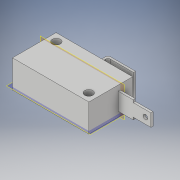
# Autodesk Inventor part: game-switch
Saved by Autodesk Inventor 2017 (Build 210142000, 142)
## iProperties
Created: 2017-02-21
Part Number: game-switch
Material: Generic
Document SubType Name: Modeling
Designer: John
Density: 1 g/cm^3
Appearance: Default
Author: John
Autodesk Inventor part; units mm, degrees
ref_plane "YZ Plane" through (0, 0, 0) normal (1, 0, 0) x (0, 1, 0)
ref_plane "XZ Plane" through (0, 0, 0) normal (0, 1, 0) x (-1, 0, 0)
sketch "Sketch1" plane through (0, 0, 0) normal (0, 1, 0) x (-1, 0, 0)
  line L0 (0, 0) -> (-28, 0)
  line L1 (-28, 0) -> (-28, 16)
  line L2 (-28, 16) -> (0, 16)
  line L3 (0, 16) -> (0, 0)
  circle A0 centre (-25.1, 13.15) radius 1.5
  circle A1 centre (-2.9, 2.85) radius 1.5
  line L4 (-28, 8) -> (0, 8) construction
  line L5 (-14, 0) -> (-14, 16) construction
  line L6 (-25.1, 13.15) -> (-28, 13.15) construction
  line L7 (-25.1, 13.15) -> (-25.1, 16) construction
  line L8 (-2.9, 2.85) -> (-2.9, 0) construction
  line L9 (-2.9, 2.85) -> (0, 2.85) construction
  dimension "d0" = 28
  dimension "d1" = 16
  dimension "d2" = 3
  dimension "d3" = 3
  dimension "d4" = 22.2
  dimension "d5" = 10.3
  constraints: 20 end point, 5 perpendicular, 4 midpoint, 4 parallel, 4 point on line, 2 centre point, 1 horizontal
  measures "d0" distance of L1.end L2.end
  measures "d1" distance of L0.end L1.end
  measures "d2" diameter of A0
  measures "d3" diameter of A1
  measures "d4" horizontal distance of L6.start L8.start
  measures "d5" vertical distance of L8.start L6.start
extrude "Extrusion1" add sketch "Sketch1" along normal blind 10.2
ref_plane "Work Plane1" through (0, 0, 4.5) normal (0, 0, 1) x (1, 0, 0)
sketch "Sketch2" plane through (0, 0, 4.5) normal (0, 0, 1) x (1, 0, 0)
  line L0 (28, 1.925) -> (33.5, 1.925)
  line L1 (33.5, 1.925) -> (33.5, 2.8)
  line L2 (33.5, 8.275) -> (28, 8.275)
  line L3 (28, 8.275) -> (28, 1.925)
  line L4 (33.5, 7.4) -> (40, 7.4)
  line L5 (40, 7.4) -> (40, 2.8)
  line L6 (40, 2.8) -> (33.5, 2.8)
  line L7 (33.5, 7.4) -> (33.5, 8.275)
  line L8 (33.5, 2.8) -> (33.5, 7.4) construction
  line L9 (28, 1.925) -> (28, 0) construction
  line L10 (28, 8.275) -> (28, 10.2) construction
  circle A0 centre (38, 5.1) radius 0.85
  line L11 (38, 5.1) -> (38, 2.8) construction
  line L12 (38, 7.4) -> (38, 5.1) construction
  point P0 (0, 0)
  dimension "d12" = 6.5
  dimension "d13" = 1.7
  dimension "d14" = 2
  dimension "d15" = 12
  dimension "d16" = 4.6
  dimension "d17" = 6.35
  constraints: 26 end point, 5 collinear, 5 parallel, 5 perpendicular, 3 point on line, 2 horizontal, 1 centre point
  measures "d12" distance of L4.start L4.end
  measures "d13" diameter of A0
  measures "d14" distance from line of L5 L11.start
  measures "d15" distance between parallel lines of L3 L5
  measures "d16" distance of L4.end L5.end
  measures "d17" distance of L2.end L0.start
extrude "Extrusion2" add sketch "Sketch2" along normal blind 0.8
ref_plane "Work Plane2" through (0, 1, 0) normal (0, -1, 0) x (1, 0, 0)
sketch "Sketch4" plane through (0, 1, 0) normal (0, -1, 0) x (1, 0, 0)
  line L0 (16.8061, 0) -> (16, 0)
  line L1 (16, 0) -> (16, -2.2)
  line L2 (16.8, -3) -> (16.8, -3)
  line L3 (16.8, -3) -> (26.1061, -3)
  line L4 (26.1061, -3) -> (26.1061, -2.2)
  line L5 (26.1061, -2.2) -> (17.6061, -2.2)
  line L6 (16.8061, -1.4) -> (16.8061, 0)
  arc A0 (16, -2.2) -> (16.8, -3) centre (16.8, -2.2) ccw
  arc A1 (16.8061, -1.4) -> (17.6061, -2.2) centre (17.6061, -1.4) ccw
  line L7 (0, 0) -> (0, 16) projected
  point P0 (16, -3)
  point P1 (16.8061, -2.2)
  dimension "d32" = 0.8
  dimension "d33" = 3
  dimension "d34" = 9.3
  dimension "d35" = 0.8
  dimension "d36" = 0.8
  dimension "d41" = 16
  constraints: 14 end point, 4 point on circle, 4 point on line, 4 tangent, 3 parallel, 2 centre point, 2 horizontal, 2 perpendicular, 1 equal radius
  measures "d32" distance of L2.end point (16, -3)
  measures "d33" distance of point (16, -3) L0.end
  measures "d34" distance of point (16.806, -2.2) L4.end
  measures "d35" distance of L4.end L3.end
  measures "d36" radius of A0
  measures "d41" distance between parallel lines of L7 L1
extrude "Extrusion3" add sketch "Sketch4" against normal blind 8.5
body "Solid1"
